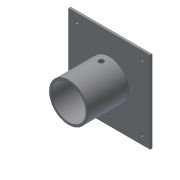
# Autodesk Inventor part: Wind Trubin Turbine Base
Saved by Autodesk Inventor 2015 SP1 (Build 190203100, 203)
## iProperties
Created: 2015-11-14
Part Number: Wind Trubin Turbine Base
Material: 一般
Document SubType Name: Modeling
Designer: nobuhiro
Density: 1 g/cm^3
Appearance: 既定
Author: nobuhiro
Autodesk Inventor part; units mm, degrees
ref_plane "YZ Plane" through (0, 0, 0) normal (1, 0, 0) x (0, 1, 0)
ref_plane "XZ Plane" through (0, 0, 0) normal (0, 1, 0) x (-1, 0, 0)
ref_plane "XY Plane" through (0, 0, 0) normal (0, 0, 1) x (1, 0, 0)
sketch "スケッチ1" plane through (0, 0, 0) normal (0, 0, 1) x (1, 0, 0)
  line L0 (0, 0) -> (0, -111.3423) construction
  line L1 (-42.5, 0) -> (-47.5, 0)
  line L2 (-47.5, 0) -> (-47.5, -105)
  line L3 (-47.5, -105) -> (-42.5, -105)
  line L4 (-42.5, -105) -> (-42.5, 0)
  dimension "d0" = 105
  dimension "d1" = 5
  dimension "d2" = 47.5
  constraints: 10 end point, 2 parallel, 1 horizontal, 1 horizontal alignment, 1 perpendicular, 1 vertical
  measures "d0" distance of L1.end L2.end
  measures "d1" distance between parallel lines of L2 L4
  measures "d2" distance between parallel lines of L0 L2
revolve "回転1" add sketch "スケッチ1" angle 360 about axis through (0, 0, 0) along (0, -1, 0)
sketch "スケッチ2" plane through (0, 0, 0) normal (0, 1, 0) x (1, 0, 0)
  circle A0 centre (0, 0) radius 42.5 projected
  line L0 (100, 100) -> (-100, 100)
  line L1 (-100, 100) -> (-100, -100)
  line L2 (-100, -100) -> (100, -100)
  line L3 (100, -100) -> (100, 100)
  line L4 (100, 100) -> (-100, -100) construction
  line L5 (-100, 100) -> (100, -100) construction
  circle A1 centre (80, -80) radius 4
  circle A2 centre (80, 80) radius 4
  circle A3 centre (-80, 80) radius 4
  circle A4 centre (-80, -80) radius 4
  dimension "d4" = 200
  dimension "d7" = 8
  dimension "d8" = 20
  dimension "d11" = 360
  constraints: 12 end point, 4 centre point, 2 midpoint, 2 parallel, 2 perpendicular, 1 horizontal, 1 point on line, 9 other
  measures "d4" distance of L1.end L2.end
  measures "d7" diameter of A1
  measures "d8" distance from line of L2 A1.centre
extrude "押し出し1" add sketch "スケッチ2" against normal blind 5 contours A0 | L3 L2 L1 L0
sketch "スケッチ3" plane through (0, 0, 0) normal (0, 0, 1) x (1, 0, 0)
  circle A0 centre (0, -25) radius 6
  line L0 (42.5, -5) -> (-42.5, -5) projected
  point P0 (0, 0)
  dimension "d13" = 12
  dimension "d14" = 20
  constraints: 1 centre point, 1 vertical alignment
  measures "d13" diameter of A0
  measures "d14" distance from line of A0.centre L0
extrude "押し出し2" cut sketch "スケッチ3" along normal through all both and the other way through all
